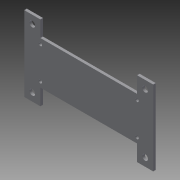
# Autodesk Inventor part: Pneumatic Piston Bracket_v1
Saved by Autodesk Inventor 2013 (Build 170138000, 138)
## iProperties
Created: 2013-01-21
Part Number: Pneumatic Piston Bracket_v1
Material: Generic
Document SubType Name: Sheet Metal
Designer: motoennies
Density: 1 g/cm^3
Sheet Metal Rule: Default
Author: motoennies
Autodesk Inventor part; units mm, degrees
ref_plane "YZ Plane" through (0, 0, 0) normal (1, 0, 0) x (0, 1, 0)
ref_plane "XZ Plane" through (0, 0, 0) normal (0, 1, 0) x (-1, 0, 0)
ref_plane "XY Plane" through (0, 0, 0) normal (0, 0, 1) x (1, 0, 0)
sketch "Sketch1" plane through (0, 0, 0) normal (0, 0, 1) x (1, 0, 0)
  line L0 (0, 50.8) -> (0, 0)
  line L1 (152.4, 0) -> (152.4, 0)
  line L2 (19.05, 0) -> (133.35, 0)
  line L3 (152.4, 0) -> (152.4, 50.8)
  line L4 (19.05, 50.8) -> (133.35, 50.8)
  line L5 (0, 50.8) -> (0, 69.85)
  line L6 (0, 69.85) -> (19.05, 69.85)
  line L7 (19.05, 69.85) -> (19.05, 50.8)
  line L8 (0, 0) -> (0, -19.05)
  line L9 (0, -19.05) -> (19.05, -19.05)
  line L10 (19.05, -19.05) -> (19.05, 0)
  line L11 (133.35, 50.8) -> (133.35, 69.85)
  line L12 (133.35, 69.85) -> (152.4, 69.85)
  line L13 (152.4, 69.85) -> (152.4, 50.8)
  line L14 (152.4, 0) -> (152.4, -19.05)
  line L15 (152.4, -19.05) -> (133.35, -19.05)
  line L16 (133.35, -19.05) -> (133.35, 0)
  dimension "d23" = 50.8
  dimension "d26" = 152.4
  dimension "d77" = 19.05
  dimension "d78" = 19.05
  dimension "d79" = 19.05
  dimension "d81" = 19.05
  dimension "d82" = 19.05
  dimension "d83" = 19.05
  dimension "d84" = 19.05
  measures "d23" distance of L0.start L0.end
  measures "d26" distance of L0.end L1.end
  measures "d77" distance of L0.start L5.end
  measures "d78" distance of L5.end L6.end
  measures "d79" distance of L0.end L8.end
  measures "d81" distance of L4.end L11.end
  measures "d82" distance of L1.end L14.end
  measures "d83" distance of L14.end L15.end
  measures "d84" distance of L11.end L12.end
extrude "Plate2" add sketch "Sketch1" along normal blind 3.048
sketch "Sketch8" plane through (0, 0, 3.048) normal (0, 0, 1) x (1, 0, 0)
  line L0 (133.35, 0) -> (19.05, 0) projected
  line L1 (19.05, 50.8) -> (19.05, 0)
  line L2 (19.05, 25.4) -> (19.05, 44.45)
  line L3 (19.05, 25.4) -> (19.05, 6.35)
  circle A0 centre (19.05, 44.45) radius 1.9844
  circle A1 centre (19.05, 6.35) radius 1.9844
  line L4 (152.4, 69.85) -> (152.4, -19.05) projected
  circle A2 centre (133.35, 44.45) radius 1.9812
  circle A3 centre (133.35, 6.35) radius 1.9812
  line L5 (19.05, -19.05) -> (0, -19.05) projected
  line L6 (19.05, 0) -> (19.05, -19.05) projected
  line L7 (133.35, -19.05) -> (133.35, 0) projected
  line L8 (152.4, -19.05) -> (133.35, -19.05) projected
  line L9 (133.35, 69.85) -> (152.4, 69.85) projected
  line L10 (19.05, 69.85) -> (19.05, 50.8) projected
  line L11 (0, 69.85) -> (19.05, 69.85) projected
  circle A4 centre (9.525, 60.325) radius 3.3782
  circle A5 centre (9.525, -9.525) radius 3.3782
  circle A6 centre (142.875, 60.325) radius 3.3782
  circle A7 centre (142.875, -9.525) radius 3.3782
  point P0 (0, 0)
  point P1 (152.4, 0)
  point P2 (152.4, 50.8)
  dimension "d63" = 19.05
  dimension "d64" = 19.05
  dimension "d65" = 3.9688
  dimension "d66" = 3.9688
  dimension "d69" = 3.9624
  dimension "d70" = 3.9624
  dimension "d71" = 19.05
  dimension "d72" = 38.1
  dimension "d73" = 19.05
  dimension "d74" = 6.35
  dimension "d85" = 6.7564
  dimension "d86" = 6.7564
  dimension "d87" = 9.525
  dimension "d88" = 9.525
  dimension "d89" = 9.525
  dimension "d90" = 9.525
  dimension "d92" = 6.7564
  dimension "d93" = 6.7564
  dimension "d94" = 9.525
  dimension "d95" = 9.525
  dimension "d96" = 9.525
  dimension "d97" = 9.525
  dimension "d98" = 6.35
  constraints: 8 centre point, 7 end point, 2 coincident, 2 point on line, 1 midpoint, 1 perpendicular
  measures "d63" distance of L2.start L2.end
  measures "d64" distance of L2.start L3.end
  measures "d65" diameter of A0
  measures "d66" diameter of A1
  measures "d69" diameter of A2
  measures "d70" diameter of A3
  measures "d71" distance from line of L4 A2.centre
  measures "d72" distance of A2.centre A3.centre
  measures "d73" distance from line of L4 A3.centre
  measures "d74" distance from line of L0 A3.centre
  measures "d85" diameter of A4
  measures "d86" diameter of A5
  measures "d87" distance from line of L11 A4.centre
  measures "d88" distance from line of L10 A4.centre
  measures "d89" distance from line of L6 A5.centre
  measures "d90" distance from line of A5.centre L5
  measures "d92" diameter of A6
  measures "d93" diameter of A7
  measures "d94" distance from line of L7 A7.centre
  measures "d95" distance from line of L8 A7.centre
  measures "d96" distance from line of L9 A6.centre
  measures "d97" distance from line of L4 A6.centre
  measures "d98" distance of L1.start A0.centre
extrude "Cut9" cut sketch "Sketch8" against normal blind 3.048
equation "\"d105\" = Thickness"
equation "\"BendRadius\" = Thickness"
equation "\"BendReliefWidth\" = Thickness"
equation "\"BendReliefDepth\" = 0.5 * Thickness"
equation "\"CornerReliefSize\" = 4 * Thickness"
equation "\"MinimumRemnant\" = 2 * Thickness"
equation "\"TransitionRadius\" = BendRadius"
equation "\"JacobiRadiusSize\" = BendRadius"
equation "\"GapSize\" = Thickness"
equation "\"d10\" = BendRadius"
equation "\"d11\" = BendRadius"
equation "\"Thickness\" = 3.048"
body "Solid2"
